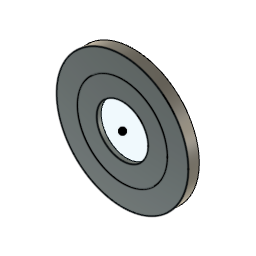
TrailerTapWasher v3 (Autodesk Fusion 360 design; units mm, degrees)
Autodesk Fusion 360 part; units mm, degrees
sketch "Sketch1" plane through (0, 0, 0) normal (0, 1, 0) x (1, 0, 0)
  circle A0 centre (0, 0) radius 11.75
  circle A1 centre (0, 0) radius 30
  circle A2 centre (0, 0) radius 20.5
  dimension "d1" = 23.5
  dimension "d2" = 60
  dimension "d3" = 41
  constraint coincident A0.centre A1.centre
  constraint concentric A0 A1
  measures "d1" diameter of A0
  measures "d2" diameter of A1
  measures "d3" diameter of A2
extrude "Extrude1" add sketch "Sketch1" along normal blind 2 contours A1 | A2
extrude "Extrude2" add sketch "Sketch1" along normal blind 5 contours A1
chamfer "Chamfer1" distance 2 angle 45 1 edges at (-19.1127, 5, -7.4131)
named bodies: "TrailerTapWasher"
